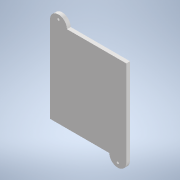
# Autodesk Inventor part: lid_arm
Saved by Autodesk Inventor 2021 (Build 250183000, 183)
## iProperties
Created: 2021-12-14
Part Number: lid_arm
Material: Generic
Document SubType Name: Modeling
Designer: marcin
Density: 1 g/cm^3
Appearance: Default
Author: marcin
Autodesk Inventor part; units mm, degrees
ref_plane "YZ Plane" through (0, 0, 0) normal (1, 0, 0) x (0, 1, 0)
ref_plane "XZ Plane" through (0, 0, 0) normal (0, 1, 0) x (-1, 0, 0)
ref_plane "XY Plane" through (0, 0, 0) normal (0, 0, 1) x (1, 0, 0)
sketch "Sketch1" plane through (0, 0, 0) normal (0, 0, 1) x (1, 0, 0)
  line L0 (40.455, 45.635) -> (-22.455, 45.635) projected
  arc A0 (-22.455, 45.635) -> (-40.455, 45.635) centre (-31.455, 45.635) ccw projected
  line L1 (-40.455, 45.635) -> (-40.455, -45.635) projected
  line L2 (-40.455, -45.635) -> (22.455, -45.635) projected
  arc A1 (22.455, -45.635) -> (40.455, -45.635) centre (31.455, -45.635) ccw projected
  line L3 (40.455, -45.635) -> (40.455, 45.635) projected
  circle A2 centre (31.455, -50.135) radius 1.15 projected
  circle A3 centre (-31.455, 50.135) radius 1.15 projected
  line L4 (-37.455, -42.635) -> (-37.455, 42.635) projected
  line L5 (-37.455, 42.635) -> (37.455, 42.635) projected
  line L6 (37.455, 42.635) -> (37.455, -42.635) projected
  line L7 (37.455, -42.635) -> (-37.455, -42.635) projected
  point P0 (0, 0)
extrude "Extrusion1" add sketch "Sketch1" along normal blind 4 contours L3 A1 L2 L1 A0 L0 | L4 L5 L6 L7
sketch "Sketch2" plane through (0, 0, 0) normal (0, 0, -1) x (-1, 0, 0)
  line L0 (37.455, 42.635) -> (37.455, -42.635) projected
  line L1 (-37.455, 42.635) -> (37.455, 42.635) projected
  line L2 (-37.455, 42.635) -> (-37.455, -42.635) projected
  line L3 (-37.455, -42.635) -> (37.455, -42.635) projected
  line L4 (37.255, -42.435) -> (37.255, 42.435)
  line L5 (37.255, 42.435) -> (-37.255, 42.435)
  line L6 (-37.255, 42.435) -> (-37.255, -42.435)
  line L7 (-37.255, -42.435) -> (37.255, -42.435)
  line L8 (34.255, 39.435) -> (34.255, -39.435)
  line L9 (34.255, -39.435) -> (-34.255, -39.435)
  line L10 (-34.255, -39.435) -> (-34.255, 39.435)
  line L11 (-34.255, 39.435) -> (34.255, 39.435)
  point P0 (0, 0)
  dimension "d2" = 0.2
  dimension "d3" = 3
  constraints: 16 end point, 6 other
  measures "d2" distance between parallel lines of L0 L4
  measures "d3" distance between parallel lines of L4 L8
extrude "Extrusion2" add sketch "Sketch2" along normal blind 3 contours L7 L6 L5 L4
body "Solid1"
